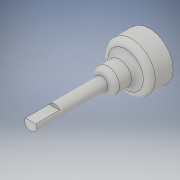
# Autodesk Inventor part: FlapperSlapper
Saved by Autodesk Inventor 2017 (Build 210142000, 142)
## iProperties
Created: 2017-10-27
Part Number: FlapperSlapper
Material: Generic
Document SubType Name: Modeling
Designer: User
Density: 1 g/cm^3
Appearance: Default
Author: User
Autodesk Inventor part; units mm, degrees
ref_plane "YZ Plane" through (0, 0, 0) normal (1, 0, 0) x (0, 1, 0)
ref_plane "XZ Plane" through (0, 0, 0) normal (0, 1, 0) x (-1, 0, 0)
ref_plane "XY Plane" through (0, 0, 0) normal (0, 0, 1) x (1, 0, 0)
sketch "Sketch1" plane through (0, 0, 0) normal (0, 0, 1) x (1, 0, 0)
  circle A0 centre (0, 0) radius 12.7
  circle A1 centre (0, 0) radius 6.35
  dimension "d0" = 25.4
  dimension "d1" = 12.7
  constraints: 2 centre point, 2 coincident
  measures "d0" diameter of A0
  measures "d1" diameter of A1
extrude "Extrusion1" add sketch "Sketch1" along normal blind 12.7
extrude "Extrusion2" add sketch "Sketch1" along normal blind 25.4 contours A1
fillet "Fillet1" radius 3.175 1 edges at (-6.35, 0, 12.7)
fillet "Fillet2" radius 3.175 1 edges at (-6.35, 0, 25.4)
sketch "Sketch2" plane through (0, 0, 12.7) normal (0, 0, 1) x (1, 0, 0)
  circle A0 centre (0, 0) radius 3.175 projected
  line L0 (0, -3.175) -> (-3.175, 0)
  line L1 (0, 3.175) -> (-3.175, 0)
  line L2 (0, 3.175) -> (3.175, 0)
  line L3 (3.175, 0) -> (0, -3.175)
  constraints: 8 end point, 3 perpendicular, 3 point on circle, 1 coincident, 1 point on line
sketch "Sketch3" plane through (0, 0, 25.4) normal (0, 0, 1) x (1, 0, 0)
  circle A0 centre (0, 0) radius 3.175
  dimension "d8" = 6.35
  constraints: 1 centre point, 1 coincident
  measures "d8" diameter of A0
extrude "Extrusion3" add sketch "Sketch3" along normal blind 266.7
sketch "Sketch4" plane through (0, 0, 292.1) normal (0, 0, 1) x (1, 0, 0)
  line L0 (0, 0) -> (0, 1.5875)
  line L1 (0, 1.5875) -> (2.7496, 1.5875)
  circle A0 centre (0, 0) radius 3.175 projected
  line L2 (0, 1.5875) -> (-2.7496, 1.5875)
  dimension "d11" = 1.5875
  constraints: 6 end point, 2 point on circle, 1 perpendicular, 1 point on line, 1 vertical
  measures "d11" distance of L0.start L0.end
extrude "Extrusion4" cut sketch "Sketch4" against normal blind 114.3 contours L2 A0 L1 picked at (-1.6863, 1.7846)
fillet "Fillet3" radius 3.175 1 edges at (-12.7, 0, 12.7)
sketch "Sketch6" plane through (0, 0, 0) normal (0, 0, -1) x (-1, 0, 0)
  circle A0 centre (0, 0) radius 2.3813
  dimension "d18" = 4.7625
  constraints: 1 centre point, 1 coincident
  measures "d18" diameter of A0
extrude "Extrusion6" cut sketch "Sketch6" against normal blind 1.5875
sketch "Sketch7" plane through (-2.7496, 1.5875, 292.1) normal (0, 1, 0) x (1, 0, 0)
  line L0 (-0.4254, 0) -> (5.9246, 0) projected
  point P0 (2.7496, 292.1)
  point P1 (2.7496, 0)
  point P2 (0, 0)
  point P3 (5.4993, 0)
  point P4 (2.7496, 8.89)
  constraints: 1 midpoint
hole "Hole1" at (0, 1.5875, 283.21) direction (0, -1, 0) diameter 3.175 depth 25.4 tip angle 118
sketch "Sketch8" plane through (-2.7496, 1.5875, 292.1) normal (0, 1, 0) x (1, 0, 0)
  line L0 (5.4993, 114.3) -> (0, 114.3) projected
  line L1 (5.4993, 114.3) -> (5.4993, 0) projected
  line L2 (0, 114.3) -> (5.4993, 114.3)
  line L3 (5.4993, 114.3) -> (5.4993, 110.49)
  line L4 (5.4993, 110.49) -> (0, 110.49)
  line L5 (0, 110.49) -> (0, 114.3)
  point P0 (2.7496, 292.1)
  dimension "d32" = 3.81
  constraints: 8 end point, 2 parallel, 1 horizontal, 1 perpendicular, 1 point on line
  measures "d32" distance of L2.end L3.end
ref_plane "Work Plane3" through (3.175, 0, 25.4) normal (-1, 0, 0) x (0, -1, 0)
thicken "Thicken1" operation add thickness 228.6 both sides no extend neighbours yes toward (0, 0, -1) faces at (0.9082, 0.0531, 292.1)
thicken "Thicken2" operation add thickness 127 both sides no extend neighbours yes toward (0, 0, -1) faces at (-0.0239, 2.3066, 177.8)
body "Solid1"
